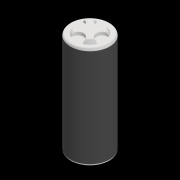
# Autodesk Inventor part: BigBattery
Saved by Autodesk Inventor 2022.1 (Build 261234000, 234)
## iProperties
Created: 2022-01-30
Part Number: BigBattery
Material: Generic
Document SubType Name: Modeling
Designer: Michael Lacey
Mass: 14.415 g
Surface Area: 37.12 cm^2
Volume: 14.415 cm^3
Density: 1 g/cm^3
Appearance: Default
Author: Michael Lacey
Autodesk Inventor part; units mm, degrees
ref_plane "YZ Plane" through (0, 0, 0) normal (1, 0, 0) x (0, 1, 0)
ref_plane "XZ Plane" through (0, 0, 0) normal (0, 1, 0) x (-1, 0, 0)
ref_plane "XY Plane" through (0, 0, 0) normal (0, 0, 1) x (1, 0, 0)
sketch "Sketch1" plane through (0, 0, 0) normal (0, 1, 0) x (-1, 0, 0)
  circle A0 centre (0, 0) radius 12.7
  dimension "d0" = 25.4
  constraints: 1 centre point, 1 coincident
  measures "d0" diameter of A0
extrude "Extrusion1" add sketch "Sketch1" along normal blind 65.8812
fillet "Fillet1" radius 1.27 2 edges at (12.7, 65.8812, 0) (12.7, 0, 0)
sketch "Sketch2" plane through (0, 65.8812, 0) normal (0, 1, 0) x (1, 0, 0)
  circle A0 centre (0, 0) radius 9.1995
  arc A1 (-8.3949, -3.7625) -> (-8.3949, 3.7625) centre (-7.9295, 0) ccw
  arc A2 (3.7625, -8.3949) -> (-3.7625, -8.3949) centre (0, -7.9295) ccw
  arc A3 (8.3949, 3.7625) -> (8.3949, -3.7625) centre (7.9295, 0) ccw
  arc A4 (-3.7625, 8.3949) -> (3.7625, 8.3949) centre (0, 7.9295) ccw
  circle A5 centre (0, 0) radius 7.9295 construction
  line L0 (-3.7625, -8.3949) -> (3.7625, -8.3949) construction
  line L1 (8.3949, -3.7625) -> (8.3949, 3.7625) construction
  line L2 (3.7625, 8.3949) -> (-3.7625, 8.3949) construction
  line L3 (-8.3949, 3.7625) -> (-8.3949, -3.7625) construction
  point P0 (3.7625, 8.3949)
  point P1 (-3.7625, 8.3949)
  point P2 (-3.7625, -8.3949)
  point P3 (3.7625, -8.3949)
  point P4 (8.3949, -3.7625)
  point P5 (8.3949, 3.7625)
  dimension "d6" = 360
  dimension "d8" = 1.27
  constraints: 13 point on circle, 8 end point, 5 centre point, 3 perpendicular, 2 coincident, 2 horizontal alignment, 1 horizontal, 19 other
extrude "Extrusion2" add sketch "Sketch2" along normal blind 2 contours A3 A0 A2 A1 A4
fillet "Fillet2" radius 2.54 4 edges at (6.5051, 67.8812, 6.5051) (-6.5051, 67.8812, 6.5051) (-6.5051, 67.8812, -6.5051) (6.5051, 67.8812, -6.5051)
body "Solid1"
